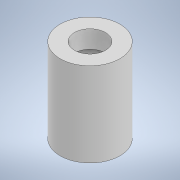
# Autodesk Inventor part: ButtonHolder_V3
Saved by Autodesk Inventor 2022.2 (Build 262287000, 287)
## iProperties
Created: 2023-03-31
Part Number: ButtonHolder_V3
Material: Generic
Document SubType Name: Modeling
Designer: jaege
Density: 1 g/cm^3
Appearance: Default
Author: jaege
Autodesk Inventor part; units mm, degrees
ref_plane "YZ Plane" through (0, 0, 0) normal (1, 0, 0) x (0, 1, 0)
ref_plane "XZ Plane" through (0, 0, 0) normal (0, 1, 0) x (-1, 0, 0)
ref_plane "XY Plane" through (0, 0, 0) normal (0, 0, 1) x (1, 0, 0)
sketch "Sketch1" plane through (0, 0, 0) normal (0, 0, 1) x (1, 0, 0)
  line L0 (0, 0) -> (4.75, 0) construction
  line L1 (6.75, 0) -> (6.75, 19)
  line L2 (6.75, 19) -> (3.5, 19)
  line L3 (3.5, 19) -> (3.5, 15)
  line L4 (3.5, 15) -> (3.5, 15)
  line L5 (3.5, 15) -> (3.5, 5) construction
  line L6 (3.5, 5) -> (0, 5) construction
  line L7 (0, 5) -> (0, 0) construction
  line L8 (4.75, 5) -> (3.5, 5)
  line L9 (3.5, 5) -> (3.5, 10.822) construction
  line L10 (3.5, 15) -> (4.75, 15)
  line L11 (4.75, 15) -> (4.75, 5)
  line L12 (4.75, 5) -> (3.5, 5)
  line L13 (4.75, 5) -> (4.75, 0)
  line L14 (4.75, 0) -> (6.75, 0)
  line L15 (0, -3.8) -> (0, 22.8) projected
  point P0 (3.375, 0)
  dimension "d0" = 4
  dimension "d7" = 3.5
  dimension "d9" = 10
  dimension "d11" = 4.75
  dimension "d12" = 2
  dimension "d13" = 5
  constraints: 30 end point, 13 perpendicular, 4 horizontal, 2 point on line, 1 coincident, 1 collinear, 1 vertical alignment
  measures "d0" distance of L2.end L3.end
  measures "d7" distance from line of L5 L6.end
  measures "d9" distance between parallel lines of L6 L4
  measures "d11" distance from line of L6.end L11
  measures "d12" distance between parallel lines of L1 L11
  measures "d13" distance between parallel lines of L0 L6
revolve "Revolution1" add sketch "Sketch1" angle 360 about axis through (0, -10, 0) along (0, 1, 0)
body "Solid1"
